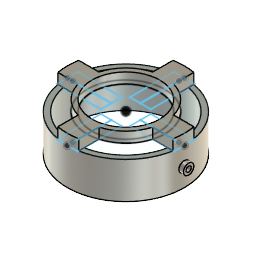
hexbug casing_revised size v2 (Autodesk Fusion 360 design; units mm, degrees)
Autodesk Fusion 360 part; units mm, degrees
sketch "Sketch1" plane through (0, 0, 0) normal (0, 0, 1) x (1, 0, 0)
  circle A0 centre (0, 0) radius 25.4
  circle A1 centre (0, 0) radius 27.94
  dimension "d1" = 50.8
  dimension "d2" = 55.88
  constraint coincident A0.centre A1.centre
  constraint concentric A0 A1
  measures "d1" diameter of A0
  measures "d2" diameter of A1
extrude "Extrude1" add sketch "Sketch1" along normal blind 17.5
sketch "Sketch2" plane through (0, 0, 17.5) normal (0, 0, 1) x (-1, 0, 0)
  circle A0 centre (0, 0) radius 25.4
  circle A1 centre (0, 0) radius 27.94
  circle A2 centre (0, 0) radius 16.15
  circle A3 centre (0, 0) radius 18.5
  line L0 (18.5, 0) -> (25.4, 0)
  line L1 (0, -18.5) -> (0, -25.4)
  line L2 (-18.5, 0) -> (-25.4, 0)
  line L3 (0, 25.4) -> (0, 18.5)
  line L4 (-27.94, 0) -> (-6.94, 0)
  line L5 (-6.94, 0) -> (-6.94, 5)
  line L6 (-6.94, 5) -> (-27.94, 5)
  line L7 (-27.94, 5) -> (-27.94, 0)
  line L8 (-27.94, 0) -> (-6.94, 0)
  line L9 (-6.94, 0) -> (-6.94, -5)
  line L10 (-6.94, -5) -> (-27.94, -5)
  line L11 (-27.94, -5) -> (-27.94, 0)
  line L12 (0, -27.94) -> (5, -27.94)
  line L13 (5, -27.94) -> (5, -6.94)
  line L14 (5, -6.94) -> (0, -6.94)
  line L15 (0, -6.94) -> (0, -27.94)
  line L16 (0, -27.94) -> (-5, -27.94)
  line L17 (-5, -27.94) -> (-5, -6.94)
  line L18 (-5, -6.94) -> (0, -6.94)
  line L19 (0, -6.94) -> (0, -27.94)
  line L20 (27.94, 0) -> (6.94, 0)
  line L21 (6.94, 0) -> (6.94, -5)
  line L22 (6.94, -5) -> (27.94, -5)
  line L23 (27.94, -5) -> (27.94, 0)
  line L24 (27.94, 0) -> (6.94, 0)
  line L25 (6.94, 0) -> (6.94, 5)
  line L26 (6.94, 5) -> (27.94, 5)
  line L27 (27.94, 5) -> (27.94, 0)
  line L28 (0, 27.94) -> (5, 27.94)
  line L29 (5, 27.94) -> (5, 6.94)
  line L30 (5, 6.94) -> (0, 6.94)
  line L31 (0, 6.94) -> (0, 27.94)
  line L32 (0, 27.94) -> (-5, 27.94)
  line L33 (-5, 27.94) -> (-5, 6.94)
  line L34 (-5, 6.94) -> (0, 6.94)
  line L35 (0, 6.94) -> (0, 27.94)
  dimension "d5" = 32.3
  dimension "d6" = 37
  dimension "d7" = 6.9
  dimension "d8" = 6.9
  dimension "d9" = 6.9
  dimension "d10" = 6.9
  dimension "d11" = 5
  dimension "d12" = 21
  dimension "d13" = 5
  dimension "d14" = 21
  dimension "d15" = 21
  dimension "d16" = 5
  dimension "d17" = 21
  dimension "d18" = 5
  dimension "d19" = 5
  dimension "d20" = 21
  dimension "d21" = 5
  dimension "d22" = 21
  dimension "d23" = 21
  dimension "d24" = 5
  dimension "d25" = 21
  dimension "d26" = 5
  constraint concentric A0 A2
  constraint concentric A0 A3
  constraint coincident A3 L0.start
  constraint coincident A0 L0.end
  constraint horizontal L0
  constraint coincident A3 L1.start
  constraint coincident A0 L1.end
  constraint perpendicular L0 L1
  constraint coincident A3 L2.start
  constraint coincident A0 L2.end
  constraint perpendicular L1 L2
  constraint coincident A0 L3.start
  constraint coincident A3 L3.end
  constraint perpendicular L2 L3
  constraint horizontal L4
  constraint vertical L5
  constraint horizontal L6
  constraint vertical L7
  constraint coincident A1 L4.start
  constraint horizontal L8
  constraint vertical L9
  constraint horizontal L10
  constraint vertical L11
  constraint horizontal L12
  constraint vertical L13
  constraint horizontal L14
  constraint vertical L15
  constraint coincident A1 L12.start
  constraint horizontal L16
  constraint vertical L17
  constraint horizontal L18
  constraint vertical L19
  constraint horizontal L20
  constraint vertical L21
  constraint horizontal L22
  constraint vertical L23
  constraint coincident A1 L20.start
  constraint horizontal L24
  constraint vertical L25
  constraint horizontal L26
  constraint vertical L27
  constraint horizontal L28
  constraint vertical L29
  constraint horizontal L30
  constraint vertical L31
  constraint coincident A1 L28.start
  constraint horizontal L32
  constraint vertical L33
  constraint horizontal L34
  constraint vertical L35
  measures "d5" diameter of A2
  measures "d6" diameter of A3
  measures "d7" distance of L2.start L2.end
  measures "d8" distance of L1.start L1.end
  measures "d9" distance of L0.start L0.end
  measures "d10" distance of L3.start L3.end
  measures "d11" distance of L4.start L6.end
  measures "d12" distance of L5.end L6.end
  measures "d13" distance of L4.start L10.end
  measures "d14" distance of L9.end L10.end
  measures "d15" distance of L12.start L14.end
  measures "d16" distance of L12.start L12.end
  measures "d17" distance of L12.start L14.end
  measures "d18" distance of L12.start L16.end
  measures "d19" distance of L20.start L22.end
  measures "d20" distance of L21.end L22.end
  measures "d21" distance of L20.start L26.end
  measures "d22" distance of L25.end L26.end
  measures "d23" distance of L28.start L30.end
  measures "d24" distance of L28.start L28.end
  measures "d25" distance of L28.start L30.end
  measures "d26" distance of L28.start L32.end
extrude "Extrude2" add sketch "Sketch2" along normal blind 5 contours A0 A3 L0 L20 L24 L26 | A0 A1 L20 L22 L24 | A0 A3 L0 L20 L22 L24 | A0 A1 L20 L24 L26 | A2 A3 L20 L24 L26 | A2 A3 L20 L22 L24 | A0 A3 L3 L29 L31 L35 | A0 A1 L29 L31 L35 | A2 A3 L26 L29 | A0 A1 L13 L15 L19 | A0 A3 L1 L13 L15 L19 | A2 A3 L13 L22 | A0 A3 L3 L31 L33 L35 | A0 A1 L31 L33 L35 | A2 A3 L29 L31 L35 | A0 A1 L15 L17 L19 | A0 A3 L1 L15 L17 L19 | A2 A3 L13 L15 L19 | A2 A3 L31 L33 L35 | A2 A3 L15 L17 L19 | A0 A3 L2 L4 L6 L8 | A0 A1 L4 L6 L8 | A2 A3 L6 L33 | A0 A1 L4 L8 L10 | A0 A3 L2 L4 L8 L10 | A2 A3 L10 L17 | A2 A3 L4 L6 L8 | A2 A3 L4 L8 L10
extrude "Extrude3" add sketch "Sketch2" along normal blind 5 contours A0 A3 L0 L20 L24 L26 | A0 A1 L20 L22 L24 | A0 A3 L0 L20 L22 L24 | A0 A1 L20 L24 L26 | A2 A3 L20 L24 L26 | A2 A3 L20 L22 L24 | A0 A3 L3 L29 L31 L35 | A0 A1 L29 L31 L35 | A2 A3 L26 L29 | A0 A1 L13 L15 L19 | A0 A3 L1 L13 L15 L19 | A2 A3 L13 L22 | A0 A3 L3 L31 L33 L35 | A0 A1 L31 L33 L35 | A2 A3 L29 L31 L35 | A0 A1 L15 L17 L19 | A0 A3 L1 L15 L17 L19 | A2 A3 L13 L15 L19 | A2 A3 L31 L33 L35 | A2 A3 L15 L17 L19 | A0 A3 L2 L4 L6 L8 | A0 A1 L4 L6 L8 | A2 A3 L6 L33 | A0 A1 L4 L8 L10 | A0 A3 L2 L4 L8 L10 | A2 A3 L10 L17 | A2 A3 L4 L6 L8 | A2 A3 L4 L8 L10
ref_plane "WorkPlane1" through (27.5, 0, 0) normal (1, 0, 0) x (0, 1, 0)
sketch "Sketch3" plane through (27.5, 0, 0) normal (1, 0, 0) x (0, 1, 0)
  line L0 (0, 0) -> (0, 17.5)
  circle A0 centre (0, 8.75) radius 1.25
  circle A1 centre (0, 8.75) radius 2.5
  dimension "d32" = 17.5
  dimension "d33" = 2.5
  dimension "d34" = 5
  constraint coincident L0.start origin
  constraint vertical L0
  constraint midpoint L0 A0.centre
  constraint concentric A0 A1
  measures "d32" distance of L0.start L0.end
  measures "d33" diameter of A0
  measures "d34" diameter of A1
extrude "Extrude4" add sketch "Sketch3" along normal blind 2.5 contours L0 A0 A1 | L0 A0 A1
